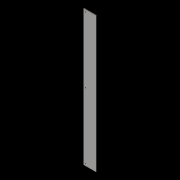
# Autodesk Inventor part: KickPlate
Saved by Autodesk Inventor 2022 (Build 260153000, 153)
## iProperties
Created: 2022-08-25
Part Number: KickPlate
Material: Steel, High Strength, Low Alloy
Document SubType Name: Modeling
Designer: tandu
Density: 7.85 g/cm^3
Appearance: Steel - Polished
Author: tandu
Autodesk Inventor part; units mm, degrees
ref_plane "YZ Plane" through (0, 0, 0) normal (1, 0, 0) x (0, 1, 0)
ref_plane "XZ Plane" through (0, 0, 0) normal (0, 1, 0) x (-1, 0, 0)
ref_plane "XY Plane" through (0, 0, 0) normal (0, 0, 1) x (1, 0, 0)
sketch "Sketch1" plane through (0, 0, 0) normal (0, 0, 1) x (1, 0, 0)
  line L0 (0, 0) -> (25.4, 0) construction
  line L1 (25.4, 0) -> (25.4, -806.45) construction
  line L2 (25.4, -806.45) -> (0, -806.45) construction
  line L3 (0, -806.45) -> (0, 0) construction
  line L4 (12.7, 0) -> (12.7, -806.45) construction
  circle A0 centre (12.7, -12.7) radius 2.5083
  circle A1 centre (12.7, -793.75) radius 2.5083
  line L5 (12.7, -12.7) -> (12.7, 0) construction
  line L6 (12.7, -12.7) -> (25.4, -12.7) construction
  line L7 (25.4, -403.225) -> (0, -403.225) construction
  line L8 (25.146, -806.196) -> (25.146, -0.254)
  line L9 (25.146, -0.254) -> (0.254, -0.254)
  line L10 (0.254, -0.254) -> (0.254, -806.196)
  line L11 (0.254, -806.196) -> (25.146, -806.196)
  line L12 (25.146, -0.254) -> (76.2, -0.254)
  line L13 (76.2, -0.254) -> (76.2, -806.196)
  line L14 (76.2, -806.196) -> (25.146, -806.196)
  circle A2 centre (12.7, -403.225) radius 2.5083
  dimension "d0" = 25.4
  dimension "d1" = 806.45
  dimension "d2" = 5.0165
  dimension "d7" = 0.254
  dimension "d8" = 50.8
  constraints: 30 end point, 5 midpoint, 4 parallel, 4 perpendicular, 3 centre point, 3 horizontal, 3 point on line, 2 equal radius, 1 collinear, 1 symmetric about line, 1 vertical, 3 other
  measures "d0" distance of L1.end L2.end
  measures "d1" distance of L0.end L1.end
  measures "d2" diameter of A0
  measures "d7" distance between parallel lines of L1 L8
  measures "d8" distance between parallel lines of L1 L13
extrude "Extrusion2" add sketch "Sketch1" along normal mid plane 3.175
fillet "Fillet2" radius 1.27 4 edges at (76.2, -0.254, 0) (0.254, -0.254, 0) (0.254, -806.196, 0) (76.2, -806.196, 0)
equation "\"d1\" = -2 * ConnectingPlateThickness + InnerLength"
equation "\"d2\" = HoleSize"
equation "\"d7\" = Tolerance"
equation "\"d9\" = ConnectingPlateThickness"
equation "\"ConnectingPlateThickness\" = 3.175"
equation "\"InnerLength\" = 812.8"
equation "\"HoleSize\" = 5.0165"
equation "\"Tolerance\" = 0.254"
body "Solid2"
